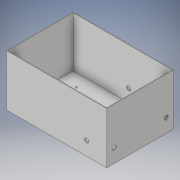
# Autodesk Inventor part: 546-1444-8-ADF4355
Saved by Autodesk Inventor 2018 (Build 220112000, 112)
## iProperties
Created: 2018-04-28
Part Number: 546-1444-8-ADF4355
Material: Generic
Document SubType Name: Modeling
Designer: bbramman
Density: 1 g/cm^3
Appearance: Default
Author: bbramman
Autodesk Inventor part; units mm, degrees
ref_plane "YZ Plane" through (0, 0, 0) normal (1, 0, 0) x (0, 1, 0)
ref_plane "XZ Plane" through (0, 0, 0) normal (0, 1, 0) x (-1, 0, 0)
ref_plane "XY Plane" through (0, 0, 0) normal (0, 0, 1) x (1, 0, 0)
sketch "Sketch1" plane through (0, 0, 0) normal (0, 1, 0) x (-1, 0, 0)
  line L0 (-76.2, 50.8) -> (76.2, 50.8)
  line L1 (76.2, 50.8) -> (76.2, -50.8)
  line L2 (76.2, -50.8) -> (-76.2, -50.8)
  line L3 (-76.2, -50.8) -> (-76.2, 50.8)
  line L4 (-76.2, 50.8) -> (76.2, -50.8) construction
  line L5 (76.2, 50.8) -> (-76.2, -50.8) construction
  point P0 (0, 0)
  dimension "d0" = 152.4
  dimension "d1" = 101.6
  constraints: 12 end point, 2 midpoint, 2 parallel, 1 horizontal, 1 perpendicular
  measures "d0" distance of L1.end L2.end
  measures "d1" distance of L0.end L1.end
extrude "Extrusion1" add sketch "Sketch1" along normal blind 2.032
sketch "Sketch2" plane through (0, 2.032, 0) normal (0, 1, 0) x (1, 0, 0)
  line L0 (-76.2, -50.8) -> (76.2, -50.8) projected
  line L1 (76.2, -50.8) -> (76.2, 50.8) projected
  line L2 (-76.2, -50.8) -> (76.2, -50.8)
  line L3 (76.2, -50.8) -> (76.2, 50.8)
  line L4 (76.2, 50.8) -> (-76.2, 50.8)
  line L5 (-76.2, 50.8) -> (-76.2, -50.8)
  line L6 (75.184, -49.784) -> (-75.184, -49.784)
  line L7 (-75.184, -49.784) -> (-75.184, 49.784)
  line L8 (-75.184, 49.784) -> (75.184, 49.784)
  line L9 (75.184, 49.784) -> (75.184, -49.784)
  line L10 (75.184, -49.784) -> (-75.184, 49.784) construction
  line L11 (-75.184, -49.784) -> (75.184, 49.784) construction
  point P0 (0, 0)
  dimension "d4" = 150.368
  dimension "d5" = 99.568
  constraints: 20 end point, 4 parallel, 2 horizontal, 2 midpoint, 2 perpendicular
  measures "d4" distance of L7.end L8.end
  measures "d5" distance of L6.end L7.end
extrude "Extrusion2" add sketch "Sketch2" along normal blind 76.2
sketch "Sketch3" plane through (0, 2.032, 0) normal (0, 1, 0) x (1, 0, 0)
  circle A0 centre (0, -25.4) radius 2.0828
  circle A1 centre (0, 25.4) radius 2.0828
  point P0 (0, 0)
  dimension "d10" = 4.1656
  dimension "d11" = 4.1656
  constraints: 2 centre point
  measures "d10" diameter of A0
  measures "d11" diameter of A1
extrude "Extrusion3" cut sketch "Sketch3" against normal through all
sketch "Sketch4" plane through (0, 2.032, 0) normal (0, 1, 0) x (1, 0, 0)
  line L0 (32.9946, -9.9949) -> (-32.9946, 9.9949) construction
  line L1 (-32.9946, -9.9949) -> (32.9946, 9.9949) construction
  circle A0 centre (-32.9946, -9.9949) radius 1.4986
  circle A1 centre (-32.9946, 9.9949) radius 1.4986
  circle A2 centre (32.9946, 9.9949) radius 1.4986
  circle A3 centre (32.9946, -9.9949) radius 1.4986
  line L2 (-70.0024, -27.7812) -> (70.0024, 27.7812) construction
  line L3 (70.0024, -27.7812) -> (-70.0024, 27.7812) construction
  circle A4 centre (34.7726, -30.3213) radius 1.5875
  circle A5 centre (34.7726, 30.3213) radius 1.5875
  circle A6 centre (-50.9524, 30.3213) radius 1.5875
  circle A7 centre (-66.8274, -30.3213) radius 1.5875
  point P0 (0, 0)
  dimension "d14" = 65.9892
  dimension "d15" = 19.9898
  dimension "d16" = 2.9972
  dimension "d17" = 2.9972
  dimension "d18" = 2.9972
  dimension "d19" = 2.9972
  dimension "d20" = 140.0048
  dimension "d21" = 55.5625
  dimension "d55" = 3.175
  dimension "d57" = 3.175
  dimension "d59" = 3.175
  dimension "d61" = 3.175
  constraints: 8 centre point, 8 end point, 4 coincident, 4 midpoint
  measures "d14" distance of L0.end L1.end
  measures "d15" distance of L1.start L0.end
  measures "d16" diameter of A0
  measures "d17" diameter of A1
  measures "d18" diameter of A2
  measures "d19" diameter of A3
  measures "d20" distance of L3.end L2.end
  measures "d21" distance of L2.end L3.start
  measures "d55" diameter of A4
  measures "d57" diameter of A5
  measures "d59" diameter of A6
  measures "d61" diameter of A7
extrude "Extrusion4" cut sketch "Sketch4" against normal through all
sketch "Sketch5" plane through (-75.184, 2.032, -49.784) normal (0, 0, 1) x (1, 0, 0)
  line L0 (151.384, 76.2) -> (-1.016, 76.2) projected
  line L1 (0.0002, 76.2) -> (150.368, 76.2)
  line L2 (150.368, 76.2) -> (150.368, 0)
  line L3 (150.368, 0) -> (0.0002, 0)
  line L4 (0.0002, 0) -> (0.0002, 76.2)
  circle A0 centre (84.5566, 19.05) radius 3.175
  circle A1 centre (100.4316, 19.05) radius 3.175
  circle A2 centre (122.6566, 19.05) radius 3.175
  point P0 (75.184, -2.032)
  dimension "d39" = 6.35
  dimension "d40" = 6.35
  dimension "d41" = 6.35
  constraints: 8 end point, 3 centre point, 2 parallel, 1 horizontal, 1 perpendicular, 1 point on line
  measures "d39" diameter of A0
  measures "d40" diameter of A1
  measures "d41" diameter of A2
extrude "Extrusion5" cut sketch "Sketch5" against normal through all contours A0 | A1 | A2
sketch "Sketch6" plane through (75.184, 2.032, -49.784) normal (-1, 0, 0) x (0, 0, 1)
  circle A0 centre (10.16, 19.05) radius 3.175
  circle A1 centre (89.408, 19.05) radius 3.175
  point P0 (49.784, -2.032)
  dimension "d44" = 6.35
  dimension "d45" = 6.35
  constraints: 2 centre point
  measures "d44" diameter of A0
  measures "d45" diameter of A1
extrude "Extrusion6" cut sketch "Sketch6" against normal through all
sketch "Sketch7" plane through (75.184, 2.032, 49.784) normal (0, 0, -1) x (-1, 0, 0)
  line L0 (150.368, 0) -> (150.368, 76.2) projected
  line L1 (150.368, 19.05) -> (155.5496, 19.05) construction
  circle A0 centre (29.2989, 19.05) radius 3.175
  point P0 (75.184, -2.032)
  dimension "d51" = 6.35
  constraints: 2 end point, 1 centre point, 1 horizontal, 1 point on line
  measures "d51" diameter of A0
extrude "Extrusion7" cut sketch "Sketch7" against normal through all
body "Solid1"
